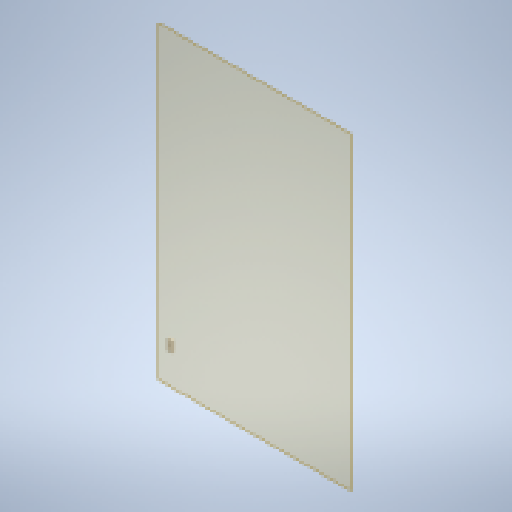
# Autodesk Inventor part: Soportes pantalla
Saved by Autodesk Inventor 2023 (Build 270158000, 158)
## iProperties
Created: 2023-05-19
Part Number: Soportes pantalla
Material: Genérico
Document SubType Name: Modeling
Designer: sergi
Density: 1 g/cm^3
Appearance: Valor por defecto
Author: sergi
Autodesk Inventor part; units mm, degrees
ref_plane "YZ Plane" through (0, 0, 0) normal (1, 0, 0) x (0, 1, 0)
ref_plane "XZ Plane" through (0, 0, 0) normal (0, 1, 0) x (-1, 0, 0)
ref_plane "XY Plane" through (0, 0, 0) normal (0, 0, 1) x (1, 0, 0)
ref_plane "Plano de trabajo1" through (0, 0, 0) normal (0, 0, 1) x (1, 0, 0)
sketch "Boceto1" plane through (0, 0, 0) normal (0, 0, 1) x (1, 0, 0)
  circle A0 centre (0.25, -2.85) radius 1.2 projected
  circle A1 centre (0.25, 2.85) radius 1.2 projected
  circle A2 centre (0.25, 309.75) radius 1.2 projected
  circle A3 centre (0.25, 304.05) radius 1.2 projected
  circle A4 centre (212.8, -3.25) radius 1.65 projected
  circle A5 centre (212.8, 5.15) radius 1.65 projected
  circle A6 centre (212.8, 310.15) radius 1.65 projected
  circle A7 centre (212.8, 301.75) radius 1.65 projected
  line L0 (-3.15, -6.55) -> (3.15, -6.55) projected
  line L1 (3.15, -6.55) -> (3.15, -26.55) projected
  line L2 (3.15, -26.55) -> (209.9, -26.55) projected
  line L3 (209.9, -26.55) -> (209.9, -6.55) projected
  line L4 (209.9, -6.55) -> (217.4, -6.55) projected
  line L5 (217.4, -6.55) -> (217.4, 8.45) projected
  line L6 (217.4, 8.45) -> (209.9, 8.45) projected
  line L7 (209.9, 8.45) -> (209.9, 11.45) projected
  line L8 (209.9, 11.45) -> (221.15, 11.45) projected
  line L9 (221.15, 11.45) -> (221.15, 295.45) projected
  line L10 (221.15, 295.45) -> (209.9, 295.45) projected
  line L11 (209.9, 295.45) -> (209.9, 298.45) projected
  line L12 (209.9, 298.45) -> (217.4, 298.45) projected
  line L13 (217.4, 298.45) -> (217.4, 313.45) projected
  line L14 (217.4, 313.45) -> (209.9, 313.45) projected
  line L15 (209.9, 313.45) -> (209.9, 333.45) projected
  line L16 (209.9, 333.45) -> (3.15, 333.45) projected
  line L17 (3.15, 333.45) -> (3.15, 313.45) projected
  line L18 (3.15, 313.45) -> (-3.15, 313.45) projected
  line L19 (-3.15, 313.45) -> (-3.15, 300.35) projected
  line L20 (-3.15, 300.35) -> (3.15, 300.35) projected
  line L21 (3.15, 300.35) -> (3.15, 6.55) projected
  line L22 (3.15, 6.55) -> (-3.15, 6.55) projected
  line L23 (-3.15, 6.55) -> (-3.15, -6.55) projected
  line L24 (3.15, 6.55) -> (3.15, -6.55)
  point P0 (0, 0)
  constraints: 2 end point, 1 vertical
extrude "Extrusión1" add sketch "Boceto1" against normal blind 3.3 contours L23 L22 L24 L0
